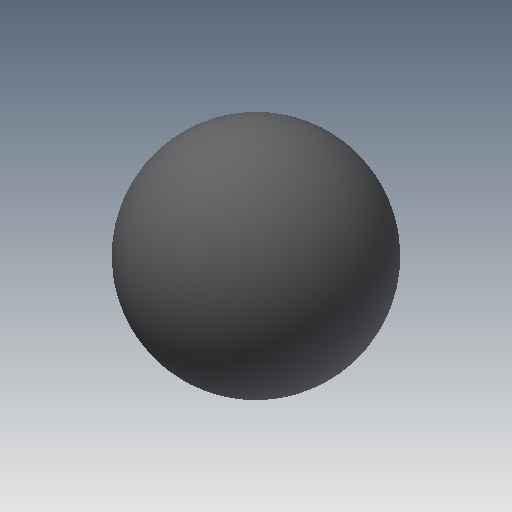
# Autodesk Inventor part: MF106ZZ1 Ball
Saved by Autodesk Inventor 2019.4 (Build 234330000, 330)
## iProperties
Category: PARTsolutions
Company: NSK_RB
Created: 2019-11-13
Part Number: MF106ZZ1 Ball
Material: 一般
Catalog Web Link: www.cadenas.de
Description: shielded_type_zz_zzs_B-
Vendor: NSK_RB
Document SubType Name: Modeling
Designer: psadmin
Manufacturer: NSK_RB
Mass: 0.000904779 g
Surface Area: 0.0452389 cm^2
Volume: 0.000904779 cm^3
Density: 1 g/cm^3
Appearance: PSOLRGB-128-128-128
PSOL_IDENT_0: {$CADENAS_DATA\23d-libs\nsk_rb\roller_bearings\deep_groove_bb\exstra_small_miniatur_bb\metric_design
PSOL_IDENT_1: _with_flange\shielded_type_zz_zzs_b_1.prj},183 {VTYP=3D},{NB=MF106ZZ1 Ball},{LINA=MF106ZZ1 Ball},{NN=
PSOL_IDENT_2: shielded_type_zz_zzs_B},{DATE=16.01.2019 01:41:14},{GEOMDATE=04.01.2008 00:00:00},{VERSION=},{LINEID=
PSOL_IDENT_3: 580},{WBVAR=},{WBNUMERIC=}  {NB=MF106ZZ1 Ball},{LINA=MF106ZZ1 Ball},{KT=DUMMY},{IDNR=},{STAN=},{ORDE
PSOL_IDENT_4: R=MF106ZZ1},{SD=6.0},{X=6.0},{D=10},{DD=10},{DD1=0.0},{D2=11.2},{DD2=11.2},{B=0.0},{B1=3.0},{CC1=0.0
PSOL_IDENT_5: },{C2=0.6},{CC2=0.6},{R=0.00},{R1=0.10},{DI1=7.00},{DI2=7.00},{SDE1=8.75},{SDE2=9.31},{CR1=495},{COR
PSOL_IDENT_6: 1=218},{CR2=51},{COR2=22.0},{LG=45000},{LO=53000},{DA=0.0},{DB=7.0},{RA=0.00},{RB=0.10},{MASS=0.77},
PSOL_IDENT_7: {SC=1}
NN: shielded_type_zz_zzs_B
NB: MF106ZZ1 Ball
NBSYN: $ORDER. Ball
LINA: MF106ZZ1 Ball
ORDER: MF106ZZ1
SD: 6
X: 6
D: 10
DD: 10
DD1: 0
D2: 11.2
DD2: 11.2
B: 0
B1: 3
CC1: 0
C2: 0.6
CC2: 0.6
R: 0
R1: 0.1
DI1: 7
DI2: 7
SDE1: 8.75
SDE2: 9.31
CR1: 495
COR1: 218
CR2: 51
COR2: 22
LG: 45000
LO: 53000
DA: 0
DB: 7
RA: 0
RB: 0.1
MASS: 0.77
SC: 1
SUPPLIER: NSK_RB
ARTICLENO: MF106ZZ1 Ball
BOMINFO: MF106ZZ1 Ball
CREATOR: CADENAS GmbH
Title: MF106ZZ1 Ball
Author: Cadenas PARTsolutions
Autodesk Inventor part; units mm, degrees
sketch "Sketch_1" plane through (0, 0, 0) normal (0, 0, 1) x (1, 0, 0)
  line L0 (0.6, 0) -> (-0.6, 0)
  arc A0 (0.6, 0) -> (-0.6, 0) centre (0, 0) ccw
  line L1 (0.6, 0) -> (-0.6, 0)
  constraints: 4 end point, 2 point on circle, 1 centre point
revolve "Revolution1" add sketch "Sketch_1" angle 360 about axis through (0.6, 0, 0) along (1, 0, 0)
ref_plane "ip_st_1_XY" through (0, 0, 0) normal (-1, 0, 0) x (0, 0, -1)
ref_plane "ip_st_1_YZ" through (0, 0, 0) normal (0, 0, -1) x (0, -1, 0)
ref_plane "ip_st_1_ZX" through (0, 0, 0) normal (0, -1, 0) x (-1, 0, 0)
body "Solid1"
